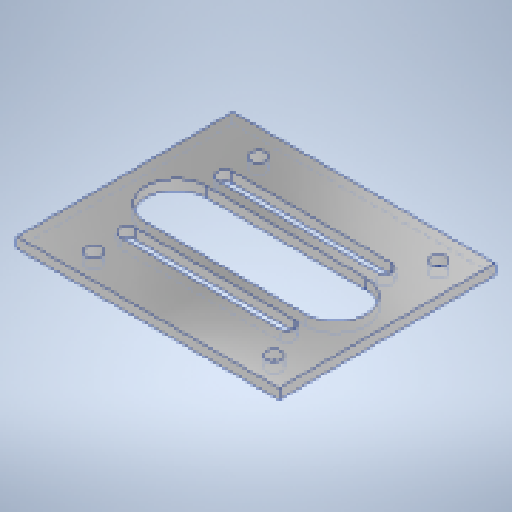
# Autodesk Inventor part: temsion1
Saved by Autodesk Inventor 2025 (Build 290162000, 162)
## iProperties
Created: 2025-03-05
Part Number: temsion1
Material: アルミニウム 6061
Document SubType Name: Modeling
Designer: Zhopa
Density: 2.7 g/cm^3
Appearance: アルミニウム - フラット
Mass: 7.71385 g
Surface Area: 37.8948 cm^2
Volume: 2.85698 cm^3
Author: Zhopa
Autodesk Inventor part; units mm, degrees
ref_plane "YZ Plane" through (0, 0, 0) normal (1, 0, 0) x (0, 1, 0)
ref_plane "XZ Plane" through (0, 0, 0) normal (0, 1, 0) x (-1, 0, 0)
ref_plane "XY Plane" through (0, 0, 0) normal (0, 0, 1) x (1, 0, 0)
sketch "Sketch1" plane through (0, 0, 0) normal (0, 1, 0) x (-1, 0, 0)
  line L0 (0, 0) -> (51, 0)
  line L1 (51, 0) -> (51, -42)
  line L2 (51, -42) -> (0, -42)
  line L3 (0, -42) -> (0, 0)
  line L4 (51, -21) -> (0, -21)
  line L5 (25.5, 0) -> (25.5, -42)
  line L6 (41, -21) -> (10, -21) construction
  line L7 (41, -15) -> (10, -15)
  line L8 (10, -27) -> (41, -27)
  arc A0 (41, -27) -> (41, -15) centre (41, -21) ccw
  arc A1 (10, -15) -> (10, -27) centre (10, -21) ccw
  line L9 (41, -30.5) -> (10, -30.5) construction
  line L10 (41, -29) -> (10, -29)
  line L11 (10, -32) -> (41, -32)
  arc A2 (41, -32) -> (41, -29) centre (41, -30.5) ccw
  arc A3 (10, -29) -> (10, -32) centre (10, -30.5) ccw
  line L12 (41, -13) -> (10, -13)
  line L13 (10, -10) -> (41, -10)
  arc A4 (41, -13) -> (41, -10) centre (41, -11.5) ccw
  arc A5 (10, -10) -> (10, -13) centre (10, -11.5) ccw
  point P0 (41, -5)
  point P1 (41, -37)
  point P2 (10, -5)
  point P3 (10, -37)
  point P4 (25.5, -21)
  point P5 (35.9893, -30.5)
  point P6 (25.5, -30.5)
  point P7 (6, -5)
  point P8 (6, -37)
  dimension "d0" = 51
  dimension "d1" = 42
  dimension "d2" = 10
  dimension "d3" = 5
  dimension "d4" = 10
  dimension "d5" = 10
  dimension "d6" = 12
  dimension "d7" = 3.5
  dimension "d8" = 3
  dimension "d18" = 6
  dimension "d19" = 6
  dimension "d20" = 3.5
  constraints: 32 end point, 12 point on circle, 9 symmetric about line, 8 tangent, 6 centre point, 6 midpoint, 4 parallel, 2 horizontal, 2 perpendicular, 2 point on line, 1 collinear, 2 other
  measures "d0" distance of L1.end L2.end
  measures "d1" distance from line of L5.end L0
  measures "d2" distance from line of L1 point (41, -5)
  measures "d3" distance from line of point (41, -5) L0
  measures "d4" distance from line of L1 L6.start
  measures "d5" distance from line of L3 L6.end
  measures "d6" diameter of A1
  measures "d7" distance from line of point (35.989, -30.5) L8
  measures "d8" diameter of A3
  measures "d18" distance from line of L3 point (6, -5)
  measures "d19" distance from line of point (6, -37) L3
  measures "d20" distance from line of L8 L9.start
extrude "Extrusion1" add sketch "Sketch1" along normal blind 2 contours L0 L5 L13 A5 L12 L7 A1 L4 L3 | L0 L1 L4 A0 L7 L5 L12 A4 L13 | L4 A1 L8 L5 L10 A3 L11 L2 L3 | L1 L2 L5 L11 A2 L10 L8 A0 L4
hole "Hole1" at (-41, 0, -5) at (-41, 0, -37) at (-41, 0, -21) at (-10, 0, -21) at (-35.9893, 0, -30.5) at (-41, 0, -30.5) at (-10, 0, -30.5) at (-41, 0, -11.5) at (-10, 0, -11.5) at (-6, 0, -5) at (-6, 0, -37) direction (0, 1, 0) diameter 3 depth 43.75 tip angle 118
equation "\"d20\" = d7"
body "Solid1"
